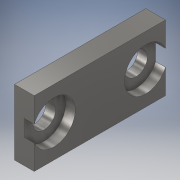
# Autodesk Inventor part: Bearing Keeper
Saved by Autodesk Inventor 2017 (Build 210142000, 142)
## iProperties
Created: 2018-11-02
Part Number: Bearing Keeper
Material: Steel, Carbon
Document SubType Name: Modeling
Designer: 623516
Density: 7.85 g/cm^3
Appearance: Semi-Polished
Author: 623516
Autodesk Inventor part; units mm, degrees
ref_plane "YZ Plane" through (0, 0, 0) normal (1, 0, 0) x (0, 1, 0)
ref_plane "XZ Plane" through (0, 0, 0) normal (0, 1, 0) x (-1, 0, 0)
ref_plane "XY Plane" through (0, 0, 0) normal (0, 0, 1) x (1, 0, 0)
sketch "Sketch1" plane through (0, 0, 0) normal (0, 1, 0) x (-1, 0, 0)
  line L0 (0, 0) -> (3, 0)
  line L1 (3, 0) -> (3, -20)
  line L2 (3, -20) -> (0, -20)
  line L3 (0, -20) -> (0, 0)
  dimension "d0" = 3
  dimension "d1" = 20
  constraints: 8 end point, 2 parallel, 1 horizontal, 1 perpendicular
  measures "d0" distance of L1.end L2.end
  measures "d1" distance of L0.end L1.end
extrude "Extrusion1" add sketch "Sketch1" along normal blind 10
sketch "Sketch2" plane through (0, 0, 0) normal (1, 0, 0) x (0, 0, -1)
  line L0 (0, 10) -> (20, 10) construction
  line L1 (10, 10) -> (10, 0) construction
  line L2 (20, 0) -> (0, 0) construction
  line L3 (10, 10) -> (3, 10) construction
  line L4 (10, 10) -> (17, 10) construction
  line L5 (10, 5) -> (0, 5) construction
  line L6 (0, 0) -> (0, 10) construction
  line L7 (10, 5) -> (20, 5) construction
  circle A0 centre (3, 5) radius 3.25 construction
  circle A1 centre (17, 5) radius 3.25 construction
  circle A2 centre (3, 5) radius 3.25
  circle A3 centre (17, 5) radius 3.25
  dimension "d4" = 7
  dimension "d5" = 7
  dimension "d6" = 6.5
  dimension "d7" = 6.5
  dimension "d8" = 6.5
  dimension "d9" = 20
  dimension "d10" = 17
  dimension "d11" = 3
  constraints: 10 end point, 4 centre point, 4 midpoint, 4 point on line, 2 coincident, 1 equal radius, 1 perpendicular
  measures "d4" distance of L1.start L3.end
  measures "d5" distance of L1.start L4.end
  measures "d6" diameter of A0
  measures "d7" diameter of A1
  measures "d8" diameter of A3
  measures "d9" distance from line of L7.end L6
  measures "d10" distance from line of A1.centre L6
  measures "d11" distance from line of A0.centre L6
extrude "Extrusion2" cut sketch "Sketch2" against normal blind 1.5
sketch "Sketch3" plane through (0, 0, 0) normal (1, 0, 0) x (0, 0, -1)
  arc A0 (0, 3.75) -> (0, 6.25) centre (3, 5) ccw construction
  line L0 (3, 1.75) -> (3, 5) construction
  arc A1 (20, 6.25) -> (20, 3.75) centre (17, 5) ccw construction
  line L1 (17, 1.75) -> (17, 5) construction
  circle A2 centre (3, 5) radius 1.75 construction
  circle A3 centre (17, 5) radius 1.75 construction
  circle A4 centre (3, 5) radius 1.75
  circle A5 centre (17, 5) radius 1.75
  point P0 (0, 0)
  dimension "d14" = 3.5
  dimension "d15" = 3.5
  constraints: 4 centre point, 4 coincident, 4 end point, 2 concentric, 2 point on circle, 2 vertical
  measures "d14" diameter of A2
  measures "d15" diameter of A3
extrude "Extrusion3" cut sketch "Sketch3" against normal blind 25374.6
body "Solid1"
